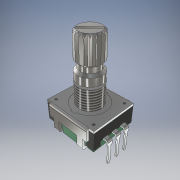
# Autodesk Inventor part: Encoder
Saved by Autodesk Inventor 2018 (Build 220112000, 112)
## iProperties
Created: 2021-02-06
Part Number: Encoder
Material: Všeobecné
Document SubType Name: Modeling
Designer: Jozko Mrkvicka
Density: 1 g/cm^3
Appearance: Výchozí
Author: Jozko Mrkvicka
Autodesk Inventor part; units mm, degrees
sketch "Náčrt1" plane through (0, 0, 0) normal (0, 1, 0) x (-1, 0, 0)
  line L0 (0, 0) -> (11.43, 0)
  line L1 (11.43, 0) -> (11.43, -13.335)
  line L2 (11.43, -13.335) -> (0, -13.335)
  line L3 (0, -13.335) -> (0, 0)
  dimension "d0" = 11.43
  dimension "d1" = 13.335
  constraints: 8 end point, 2 parallel, 1 horizontal, 1 perpendicular
  measures "d0" distance of L1.end L2.end
  measures "d1" distance of L0.end L1.end
extrude "Vysunutí1" add sketch "Náčrt1" along normal blind 3.175
sketch "Náčrt2" plane through (0, 3.175, 0) normal (0, 1, 0) x (1, 0, 0)
  line L0 (-11.43, 13.335) -> (-9.525, 13.335)
  line L1 (-9.525, 13.335) -> (-9.525, 12.7)
  line L2 (-9.525, 12.7) -> (-10.795, 12.7)
  line L3 (-10.795, 12.7) -> (-10.795, 11.43)
  line L4 (-10.795, 11.43) -> (-11.43, 11.43)
  line L5 (-11.43, 11.43) -> (-11.43, 13.335)
  line L6 (-11.43, 0) -> (-11.43, 1.905)
  line L7 (-11.43, 1.905) -> (-10.795, 1.905)
  line L8 (-10.795, 1.905) -> (-10.795, 0.635)
  line L9 (-10.795, 0.635) -> (-9.525, 0.635)
  line L10 (-9.525, 0.635) -> (-9.525, 0)
  line L11 (-9.525, 0) -> (-11.43, 0)
  line L12 (0, 0) -> (-1.905, 0)
  line L13 (-1.905, 0) -> (-1.905, 0.635)
  line L14 (-1.905, 0.635) -> (-0.635, 0.635)
  line L15 (-0.635, 0.635) -> (-0.635, 1.905)
  line L16 (-0.635, 1.905) -> (0, 1.905)
  line L17 (0, 1.905) -> (0, 0)
  line L18 (0, 13.335) -> (0, 11.43)
  line L19 (0, 11.43) -> (-0.635, 11.43)
  line L20 (-0.635, 11.43) -> (-0.635, 12.7)
  line L21 (-0.635, 12.7) -> (-1.905, 12.7)
  line L22 (-1.905, 12.7) -> (-1.905, 13.335)
  line L23 (-1.905, 13.335) -> (0, 13.335)
  point P0 (-11.43, 0)
  point P1 (0, 0)
  point P2 (0, 0)
  point P3 (0, 13.335)
  dimension "d4" = 1.905
  dimension "d5" = 0.635
  dimension "d6" = 1.27
  dimension "d7" = 1.27
  dimension "d8" = 1.905
  dimension "d9" = 0.635
  dimension "d10" = 1.27
  dimension "d11" = 1.27
  dimension "d12" = 1.905
  dimension "d13" = 0.635
  dimension "d14" = 1.27
  dimension "d15" = 1.27
  dimension "d16" = 1.905
  dimension "d17" = 0.635
  dimension "d18" = 1.27
  dimension "d19" = 1.27
  constraints: 48 end point, 8 perpendicular, 1 coincident, 1 vertical
  measures "d4" distance of L0.start L0.end
  measures "d5" distance of L0.end L1.end
  measures "d6" distance of L1.end L2.end
  measures "d7" distance of L2.end L3.end
  measures "d8" distance of L6.start L6.end
  measures "d9" distance of L6.end L7.end
  measures "d10" distance of L7.end L8.end
  measures "d11" distance of L8.end L9.end
  measures "d12" distance of L12.start L12.end
  measures "d13" distance of L12.end L13.end
  measures "d14" distance of L13.end L14.end
  measures "d15" distance of L14.end L15.end
  measures "d16" distance of L18.start L18.end
  measures "d17" distance of L18.end L19.end
  measures "d18" distance of L19.end L20.end
  measures "d19" distance of L20.end L21.end
extrude "Vysunutí2" add sketch "Náčrt2" along normal blind 1.27
sketch "Náčrt3" plane through (0, 3.175, 0) normal (0, 1, 0) x (1, 0, 0)
  line L0 (-11.43, 11.43) -> (-11.43, 1.905) projected
  line L1 (-10.795, 0.635) -> (-0.635, 0.635)
  line L2 (-0.635, 12.7) -> (-10.795, 12.7)
  line L3 (-11.43, 4.445) -> (-11.43, 8.89)
  line L4 (0, 8.89) -> (0, 4.445)
  line L5 (0, 4.445) -> (-0.635, 4.445)
  line L6 (-10.795, 4.445) -> (-11.43, 4.445)
  line L7 (-11.43, 8.89) -> (-10.795, 8.89)
  line L8 (-0.635, 8.89) -> (0, 8.89)
  line L9 (-10.795, 12.7) -> (-10.795, 8.89)
  line L10 (-10.795, 4.445) -> (-10.795, 0.635)
  line L11 (-0.635, 0.635) -> (-0.635, 4.445)
  line L12 (-0.635, 8.89) -> (-0.635, 12.7)
  point P0 (0, 0)
  point P1 (-5.715, 6.6675)
  dimension "d22" = 4.445
  constraints: 24 end point, 10 parallel, 4 perpendicular, 3 horizontal, 1 point on line
  measures "d22" distance of L3.start L3.end
extrude "Vysunutí3" add sketch "Náčrt3" along normal blind 2.54
ref_plane "Pracovní rovina1" through (-10.795, 3.175, -3.175) normal (0, 1, 0) x (1, 0, 0)
split_face "Rozdělit1"
sketch "Náčrt4" plane through (0, 5.715, 0) normal (0, 1, 0) x (1, 0, 0)
  line L0 (-0.635, 4.445) -> (-0.635, 1.905) projected
  line L1 (-0.635, 4.445) -> (-0.635, 1.905)
  line L2 (-10.795, 1.905) -> (-10.795, 4.445)
  line L3 (-10.795, 11.43) -> (-10.795, 8.89)
  line L4 (-0.635, 11.1125) -> (-0.635, 9.2075)
  line L5 (-10.795, 9.2075) -> (-10.795, 11.1125)
  line L6 (-0.635, 4.1275) -> (-0.635, 2.2225)
  line L7 (-10.795, 2.2225) -> (-10.795, 4.1275)
  line L8 (-0.635, 11.1125) -> (-2.54, 11.1125)
  line L9 (-2.54, 11.1125) -> (-2.54, 9.2075)
  line L10 (-2.54, 9.2075) -> (-0.635, 9.2075)
  line L11 (-0.635, 9.2075) -> (-0.635, 11.1125)
  line L12 (-0.635, 4.1275) -> (-2.54, 4.1275)
  line L13 (-2.54, 4.1275) -> (-2.54, 2.2225)
  line L14 (-2.54, 2.2225) -> (-0.635, 2.2225)
  line L15 (-0.635, 2.2225) -> (-0.635, 4.1275)
  line L16 (-10.795, 11.1125) -> (-8.89, 11.1125)
  line L17 (-8.89, 11.1125) -> (-8.89, 9.2075)
  line L18 (-8.89, 9.2075) -> (-10.795, 9.2075)
  line L19 (-10.795, 9.2075) -> (-10.795, 11.1125)
  line L20 (-10.795, 4.1275) -> (-8.89, 4.1275)
  line L21 (-8.89, 4.1275) -> (-8.89, 2.2225)
  line L22 (-8.89, 2.2225) -> (-10.795, 2.2225)
  line L23 (-10.795, 2.2225) -> (-10.795, 4.1275)
  point P0 (0, 0)
  point P1 (-5.715, 10.16)
  point P2 (-5.715, 3.175)
  dimension "d26" = 1.905
  dimension "d27" = 1.905
  dimension "d28" = 1.905
  dimension "d29" = 1.905
  dimension "d30" = 1.905
  dimension "d31" = 1.905
  dimension "d32" = 1.905
  constraints: 46 end point, 11 parallel, 4 horizontal, 4 perpendicular, 1 point on line
  measures "d26" distance of L4.start L4.end
  measures "d27" distance of L6.start L6.end
  measures "d28" distance of L10.end L9.end
  measures "d29" distance of L9.end L8.end
  measures "d30" distance of L14.end L13.end
  measures "d31" distance of L17.end L18.end
  measures "d32" distance of L21.end L22.end
extrude "Vysunutí4" cut sketch "Náčrt4" against normal blind 0.635
sketch "Náčrt5" plane through (0, 0, 0) normal (0, -1, 0) x (1, 0, 0)
  line L0 (0, 0) -> (-11.43, 0) projected
  line L1 (-11.43, 0) -> (-11.43, -13.335) projected
  line L2 (-11.43, -13.335) -> (0, -13.335) projected
  line L3 (0, -13.335) -> (0, 0) projected
  line L4 (0, -13.335) -> (-11.43, -13.335)
  line L5 (-11.43, 0) -> (0, 0)
  line L6 (-11.43, -12.065) -> (-12.065, -12.065)
  line L7 (-12.065, -12.065) -> (-12.065, -1.27)
  line L8 (-12.065, -1.27) -> (-11.43, -1.27)
  line L9 (0, -13.335) -> (0, -11.43) projected
  line L10 (0, -12.065) -> (0.635, -12.065)
  line L11 (0.635, -12.065) -> (0.635, -1.27)
  line L12 (0.635, -1.27) -> (0, -1.27)
  line L13 (0, 0) -> (0, -1.27)
  line L14 (0, -12.065) -> (0, -13.335)
  line L15 (-11.43, -13.335) -> (-11.43, -12.065)
  line L16 (-11.43, -1.27) -> (-11.43, 0)
  dimension "d126" = 1.27
  constraints: 24 end point, 7 parallel, 4 perpendicular, 3 horizontal, 3 point on line
  measures "d126" distance between parallel lines of L12 L0
extrude "Vysunutí5" add sketch "Náčrt5" along normal blind 0.635
ref_plane "Pracovní rovina2" through (0.3175, 0, -1.27) normal (0, 1, 0) x (1, 0, 0)
split_face "Rozdělit2"
sketch "Náčrt6" plane through (0, 0, 0) normal (0, 1, 0) x (1, 0, 0)
  line L0 (0, 1.27) -> (0, 0) projected
  line L1 (0.635, 12.065) -> (0, 12.065)
  line L2 (0, 12.065) -> (0, 1.27)
  line L3 (0, 1.27) -> (0.635, 1.27)
  line L4 (0.635, 1.27) -> (0.635, 12.065)
  line L5 (-11.43, 12.065) -> (-11.43, 13.335) projected
  line L6 (-11.43, 1.27) -> (-12.065, 1.27) projected
  line L7 (-11.43, 12.065) -> (-12.065, 12.065)
  line L8 (-12.065, 12.065) -> (-12.065, 1.27)
  line L9 (-12.065, 1.27) -> (-11.43, 1.27)
  line L10 (-11.43, 1.27) -> (-11.43, 12.065)
  constraints: 16 end point, 4 parallel, 2 horizontal, 2 perpendicular
extrude "Vysunutí6" add sketch "Náčrt6" along normal blind 2.54
sketch "Náčrt7" plane through (0, 2.54, 0) normal (0, 1, 0) x (1, 0, 0)
  line L0 (-2.54, 11.1125) -> (-0.635, 11.1125) projected
  line L1 (-0.635, 11.1125) -> (-0.635, 9.2075) projected
  line L2 (-2.54, 4.1275) -> (-0.635, 4.1275) projected
  line L3 (-0.635, 4.1275) -> (-0.635, 2.2225) projected
  line L4 (-10.795, 4.1275) -> (-8.89, 4.1275) projected
  line L5 (-8.89, 2.2225) -> (-10.795, 2.2225) projected
  line L6 (-10.795, 11.1125) -> (-8.89, 11.1125) projected
  line L7 (-8.89, 9.2075) -> (-10.795, 9.2075) projected
  line L8 (0, 9.3962) -> (0.635, 9.3962)
  line L9 (0.635, 9.3962) -> (0.635, 10.9238)
  line L10 (0.635, 10.9238) -> (0, 10.9238)
  line L11 (0, 10.9238) -> (0, 9.3962)
  line L12 (0, 9.3962) -> (0.635, 10.9238) construction
  line L13 (0.635, 9.3962) -> (0, 10.9238) construction
  line L14 (0, 2.4094) -> (0.635, 2.4094)
  line L15 (0.635, 2.4094) -> (0.635, 3.9406)
  line L16 (0.635, 3.9406) -> (0, 3.9406)
  line L17 (0, 3.9406) -> (0, 2.4094)
  line L18 (0, 2.4094) -> (0.635, 3.9406) construction
  line L19 (0.635, 2.4094) -> (0, 3.9406) construction
  line L20 (-11.43, 2.4094) -> (-12.065, 2.4094)
  line L21 (-12.065, 2.4094) -> (-12.065, 3.9406)
  line L22 (-12.065, 3.9406) -> (-11.43, 3.9406)
  line L23 (-11.43, 3.9406) -> (-11.43, 2.4094)
  line L24 (-11.43, 2.4094) -> (-12.065, 3.9406) construction
  line L25 (-12.065, 2.4094) -> (-11.43, 3.9406) construction
  line L26 (-11.43, 9.3962) -> (-12.065, 9.3962)
  line L27 (-12.065, 9.3962) -> (-12.065, 10.9238)
  line L28 (-12.065, 10.9238) -> (-11.43, 10.9238)
  line L29 (-11.43, 10.9238) -> (-11.43, 9.3962)
  line L30 (-11.43, 9.3962) -> (-12.065, 10.9238) construction
  line L31 (-12.065, 9.3962) -> (-11.43, 10.9238) construction
  point P0 (0.3175, 10.16)
  point P1 (0.3175, 3.175)
  point P2 (-11.7475, 3.175)
  point P3 (-11.7475, 10.16)
  constraints: 48 end point, 8 midpoint, 8 parallel, 4 horizontal, 4 perpendicular, 2 point on line
extrude "Vysunutí7" add sketch "Náčrt7" along normal up to surface (3.175 mm away)
sketch "Náčrt8" plane through (0, 3.175, -9.3962) normal (-1, 0, 0) x (0, 0, 1)
  line L0 (-1.5276, 0) -> (-1.5276, 2.54) projected
  line L1 (0.1887, 1.905) -> (-1.7163, 1.905) projected
  line L2 (0, 2.54) -> (-1.5276, 2.54)
  line L3 (-1.5276, 2.54) -> (-1.5276, 1.905)
  line L4 (-1.5276, 1.905) -> (0, 1.905)
  line L5 (0, 1.905) -> (0, 2.54)
  line L6 (7.1737, 1.905) -> (5.2687, 1.905) projected
  line L7 (6.9868, 2.54) -> (5.4555, 2.54) projected
  line L8 (5.4555, 0) -> (5.4555, 2.54) projected
  line L9 (6.9868, 2.54) -> (5.4555, 2.54)
  line L10 (5.4555, 2.54) -> (5.4555, 1.905)
  line L11 (5.4555, 1.905) -> (6.9868, 1.905)
  line L12 (6.9868, 1.905) -> (6.9868, 2.54)
  point P0 (9.3962, -3.175)
  constraints: 16 end point, 4 parallel, 4 point on line, 2 horizontal, 2 perpendicular
extrude "Vysunutí8" add sketch "Náčrt8" along normal blind 1.905
sketch "Náčrt9" plane through (-11.43, 3.175, -3.9406) normal (1, 0, 0) x (0, 0, -1)
  line L0 (-1.5313, 0) -> (-1.5313, 2.54) projected
  line L1 (0.1869, 1.905) -> (-1.7181, 1.905) projected
  line L2 (7.1719, 1.905) -> (5.2669, 1.905) projected
  line L3 (5.4555, 0) -> (5.4555, 2.54) projected
  line L4 (6.9832, 2.54) -> (5.4555, 2.54)
  line L5 (5.4555, 2.54) -> (5.4555, 1.905)
  line L6 (5.4555, 1.905) -> (6.9832, 1.905)
  line L7 (6.9832, 1.905) -> (6.9832, 2.54)
  line L8 (0, -0.635) -> (0, 2.54) projected
  line L9 (0, 2.54) -> (-1.5313, 2.54)
  line L10 (-1.5313, 2.54) -> (-1.5313, 1.905)
  line L11 (-1.5313, 1.905) -> (0, 1.905)
  line L12 (0, 1.905) -> (0, 2.54)
  point P0 (-3.9406, -3.175)
  constraints: 16 end point, 4 parallel, 4 point on line, 2 horizontal, 2 perpendicular
extrude "Vysunutí9" add sketch "Náčrt9" along normal blind 1.905
fillet "Zaoblení1" radius 0.635 6 edges at (-12.065, 5.715, -10.16) (-12.065, 5.715, -3.175) (0.635, 5.715, -3.175) (0.635, 5.715, -10.16) (0.635, -0.635, -6.6675) (-12.065, -0.635, -6.6675)
fillet "Zaoblení2" radius 0.3175 8 edges at (-11.43, 5.08, -3.175) (-11.43, 5.08, -10.16) (0, 5.08, -10.16) (0, 5.08, -3.175) (-9.525, 5.715, -10.16) (-9.525, 5.715, -3.175) (-1.905, 5.715, -3.175) (-1.905, 5.715, -10.16)
sketch "Náčrt10" plane through (0, -0.635, 0) normal (0, -1, 0) x (1, 0, 0)
  circle A0 centre (-10.16, -12.065) radius 0.3175
  circle A1 centre (-10.16, -1.27) radius 0.3175
  circle A2 centre (-1.27, -1.27) radius 0.3175
  circle A3 centre (-1.27, -12.065) radius 0.3175
  line L0 (-10.4775, -6.0325) -> (-10.4775, -7.3025)
  line L1 (-0.9525, -7.3025) -> (-0.9525, -6.0325)
  line L2 (-10.4775, -7.3025) -> (-10.1144, -7.3025)
  line L3 (-1.3156, -7.3025) -> (-0.9525, -7.3025)
  line L4 (-0.9525, -6.0325) -> (-1.3156, -6.0325)
  line L5 (-10.1144, -6.0325) -> (-10.4775, -6.0325)
  arc A4 (-10.1144, -7.3025) -> (-1.3156, -7.3025) centre (-5.715, -6.6675) ccw
  arc A5 (-1.3156, -6.0325) -> (-10.1144, -6.0325) centre (-5.715, -6.6675) ccw
  line L6 (-11.43, -12.065) -> (-11.43, -1.27) projected
  line L7 (-11.43, -13.335) -> (0, -13.335) projected
  line L8 (0, -13.335) -> (0, -12.065) projected
  line L9 (0, -1.27) -> (0, 0) projected
  line L10 (0, 0) -> (-11.43, 0) projected
  dimension "d55" = 0.635
  dimension "d57" = 0.635
  dimension "d59" = 9.525
  dimension "d60" = 1.27
  dimension "d118" = 1.27
  dimension "d119" = 1.27
  dimension "d120" = 1.27
  dimension "d121" = 1.27
  dimension "d122" = 1.27
  dimension "d123" = 1.27
  dimension "d124" = 1.27
  dimension "d125" = 1.27
  constraints: 12 end point, 6 centre point, 5 parallel, 4 point on circle, 2 coincident, 2 horizontal, 2 perpendicular
  measures "d55" diameter of A1
  measures "d57" diameter of A3
  measures "d59" distance of L1.start L0.end
  measures "d60" distance of L0.end L0.start
  measures "d118" distance from line of L7 point (-10.16, -12.065)
  measures "d119" distance from line of L6 point (-10.16, -12.065)
  measures "d120" distance from line of L7 A3.centre
  measures "d121" distance from line of L8 A3.centre
  measures "d122" distance from line of L10 A2.centre
  measures "d123" distance from line of L9 A2.centre
  measures "d124" distance from line of L10 point (-10.16, -1.27)
  measures "d125" distance from line of L6 point (-10.16, -1.27)
extrude "Vysunutí10" cut sketch "Náčrt10" against normal blind 0.0635
sketch "Náčrt11" plane through (0, -0.5715, 0) normal (0, -1, 0) x (1, 0, 0)
  arc A0 (-10.1144, -7.3025) -> (-1.3156, -7.3025) centre (-5.715, -6.6675) ccw projected
  circle A1 centre (-5.715, -6.6675) radius 3.175
  point P0 (0, 0)
  dimension "d63" = 6.35
  constraints: 1 centre point, 1 coincident
  measures "d63" diameter of A1
extrude "Vysunutí11" add sketch "Náčrt11" along normal blind 5.08
sketch "Náčrt12" plane through (-5.715, -5.6515, -6.6675) normal (0, -1, 0) x (1, 0, 0)
  circle A0 centre (0, 0) radius 3.175 projected
  circle A1 centre (0, 0) radius 2.2225
  point P0 (5.715, 6.6675)
  dimension "d66" = 4.445
  constraints: 1 centre point, 1 coincident
  measures "d66" diameter of A1
extrude "Vysunutí12" add sketch "Náčrt12" along normal blind 0.635 contours A1
sketch "Náčrt13" plane through (-5.715, -6.2865, -6.6675) normal (0, -1, 0) x (1, 0, 0)
  circle A0 centre (0, 0) radius 3.175 projected
  circle A1 centre (0, 0) radius 3.175
  point P0 (5.715, 6.6675)
  constraints: 1 centre point, 1 coincident
extrude "Vysunutí14" add sketch "Náčrt13" along normal blind 2.54
chamfer "Zkosení1" distance 0.635 angle 45 1 edges at (-8.89, -8.8265, -6.6675)
sketch "Náčrt14" plane through (-5.715, -8.8265, -6.6675) normal (0, -1, 0) x (1, 0, 0)
  circle A0 centre (0, 0) radius 2.54 projected
  point P0 (5.715, 6.6675)
extrude "Vysunutí15" add sketch "Náčrt14" along normal blind 1.27
sketch "Náčrt15" plane through (-5.715, -10.0965, -6.6675) normal (0, -1, 0) x (1, 0, 0)
  circle A0 centre (0, 0) radius 3.175
  point P0 (5.715, 6.6675)
  point P1 (-2.5087, 0.3973)
  point P2 (-2.5087, -0.3973)
  point P3 (-2.2632, -1.1531)
  point P4 (-2.5087, -0.3973)
  point P5 (-1.7961, -1.7961)
  point P6 (-2.2632, -1.1531)
  point P7 (-1.1531, -2.2632)
  point P8 (-1.7961, -1.7961)
  point P9 (-0.3973, -2.5087)
  point P10 (-1.1531, -2.2632)
  point P11 (0.3973, -2.5087)
  point P12 (-0.3973, -2.5087)
  point P13 (1.1531, -2.2632)
  point P14 (0.3973, -2.5087)
  point P15 (1.7961, -1.7961)
  point P16 (1.1531, -2.2632)
  point P17 (2.2632, -1.1531)
  point P18 (1.7961, -1.7961)
  point P19 (2.5087, -0.3973)
  point P20 (2.2632, -1.1531)
  point P21 (2.5087, 0.3973)
  point P22 (2.5087, -0.3973)
  point P23 (2.2632, 1.1531)
  point P24 (2.5087, 0.3973)
  point P25 (1.7961, 1.7961)
  point P26 (2.2632, 1.1531)
  point P27 (1.1531, 2.2632)
  point P28 (1.7961, 1.7961)
  point P29 (0.3973, 2.5087)
  point P30 (1.1531, 2.2632)
  point P31 (-0.3973, 2.5087)
  point P32 (0.3973, 2.5087)
  point P33 (-1.1531, 2.2632)
  point P34 (-0.3973, 2.5087)
  point P35 (-1.7961, 1.7961)
  point P36 (-1.1531, 2.2632)
  point P37 (-2.2632, 1.1531)
  point P38 (-1.7961, 1.7961)
  point P39 (-2.5087, 0.3973)
  point P40 (-2.2632, 1.1531)
  constraints: 1 centre point, 1 coincident
extrude "Vysunutí17" add sketch "Náčrt15" along normal blind 6.35
chamfer "Zkosení2" distance 0.635 angle 45 2 edges at (-8.89, -16.4465, -6.6675) (-8.89, -10.0965, -6.6675)
sketch "Náčrt16" plane through (-5.715, -16.4465, -6.6675) normal (0, -1, 0) x (1, 0, 0)
  line L0 (5.08, 6.0325) -> (3.81, 6.0325) projected
  line L1 (2.54, 0) -> (3.3297, 0.6582)
  line L2 (3.3297, 0.6582) -> (3.3297, -0.6582)
  line L3 (5.3975, 4.2581) -> (5.3975, 2.7269) projected
  line L4 (2.54, 0) -> (3.3297, -0.6582)
  line L5 (2.4157, 0.7849) -> (2.9633, 1.6549)
  line L6 (2.9633, 1.6549) -> (3.3701, 0.403)
  line L7 (2.4157, 0.7849) -> (3.3701, 0.403)
  line L8 (2.0549, 1.493) -> (2.3069, 2.4896)
  line L9 (2.3069, 2.4896) -> (3.0806, 1.4247)
  line L10 (2.0549, 1.493) -> (3.0806, 1.4247)
  line L11 (1.493, 2.0549) -> (1.4247, 3.0806)
  line L12 (1.4247, 3.0806) -> (2.4896, 2.3069)
  line L13 (1.493, 2.0549) -> (2.4896, 2.3069)
  line L14 (0.7849, 2.4157) -> (0.403, 3.3701)
  line L15 (0.403, 3.3701) -> (1.6549, 2.9633)
  line L16 (0.7849, 2.4157) -> (1.6549, 2.9633)
  line L17 (0, 2.54) -> (-0.6582, 3.3297)
  line L18 (-0.6582, 3.3297) -> (0.6582, 3.3297)
  line L19 (0, 2.54) -> (0.6582, 3.3297)
  line L20 (-0.7849, 2.4157) -> (-1.6549, 2.9633)
  line L21 (-1.6549, 2.9633) -> (-0.403, 3.3701)
  line L22 (-0.7849, 2.4157) -> (-0.403, 3.3701)
  line L23 (-1.493, 2.0549) -> (-2.4896, 2.3069)
  line L24 (-2.4896, 2.3069) -> (-1.4247, 3.0806)
  line L25 (-1.493, 2.0549) -> (-1.4247, 3.0806)
  line L26 (-2.0549, 1.493) -> (-3.0806, 1.4247)
  line L27 (-3.0806, 1.4247) -> (-2.3069, 2.4896)
  line L28 (-2.0549, 1.493) -> (-2.3069, 2.4896)
  line L29 (-2.4157, 0.7849) -> (-3.3701, 0.403)
  line L30 (-3.3701, 0.403) -> (-2.9633, 1.6549)
  line L31 (-2.4157, 0.7849) -> (-2.9633, 1.6549)
  line L32 (-2.54, 0) -> (-3.3297, -0.6582)
  line L33 (-3.3297, -0.6582) -> (-3.3297, 0.6582)
  line L34 (-2.54, 0) -> (-3.3297, 0.6582)
  line L35 (-2.4157, -0.7849) -> (-2.9633, -1.6549)
  line L36 (-2.9633, -1.6549) -> (-3.3701, -0.403)
  line L37 (-2.4157, -0.7849) -> (-3.3701, -0.403)
  line L38 (-2.0549, -1.493) -> (-2.3069, -2.4896)
  line L39 (-2.3069, -2.4896) -> (-3.0806, -1.4247)
  line L40 (-2.0549, -1.493) -> (-3.0806, -1.4247)
  line L41 (-1.493, -2.0549) -> (-1.4247, -3.0806)
  line L42 (-1.4247, -3.0806) -> (-2.4896, -2.3069)
  line L43 (-1.493, -2.0549) -> (-2.4896, -2.3069)
  line L44 (-0.7849, -2.4157) -> (-0.403, -3.3701)
  line L45 (-0.403, -3.3701) -> (-1.6549, -2.9633)
  line L46 (-0.7849, -2.4157) -> (-1.6549, -2.9633)
  line L47 (0, -2.54) -> (0.6582, -3.3297)
  line L48 (0.6582, -3.3297) -> (-0.6582, -3.3297)
  line L49 (0, -2.54) -> (-0.6582, -3.3297)
  line L50 (0.7849, -2.4157) -> (1.6549, -2.9633)
  line L51 (1.6549, -2.9633) -> (0.403, -3.3701)
  line L52 (0.7849, -2.4157) -> (0.403, -3.3701)
  line L53 (1.493, -2.0549) -> (2.4896, -2.3069)
  line L54 (2.4896, -2.3069) -> (1.4247, -3.0806)
  line L55 (1.493, -2.0549) -> (1.4247, -3.0806)
  line L56 (2.0549, -1.493) -> (3.0806, -1.4247)
  line L57 (3.0806, -1.4247) -> (2.3069, -2.4896)
  line L58 (2.0549, -1.493) -> (2.3069, -2.4896)
  line L59 (2.4157, -0.7849) -> (3.3701, -0.403)
  line L60 (3.3701, -0.403) -> (2.9633, -1.6549)
  line L61 (2.4157, -0.7849) -> (2.9633, -1.6549)
  point P0 (0, 0)
  point P1 (5.715, 6.6675)
  point P2 (0, 0)
  dimension "d113" = 360
  constraints: 120 end point, 1 coincident, 1 parallel, 121 other
extrude "Vysunutí18" cut sketch "Náčrt16" against normal blind 6.35 contours L1 L7 L2 L59 L4 | L7 L5 L10 L6 L1 | L1 L6 L2 L7 | L59 L2 L60 L4 | L4 L60 L56 L61 L59 | L1 L2 L6 | L2 L6 L7 | L60 L2 L4 | L59 L60 L2 | L10 L5 L9 L6 | L6 L9 L10 | L10 L8 L13 L9 L5 | L60 L57 L61 L56 | L56 L57 L60 | L61 L57 L53 L58 L56 | L9 L5 L6 | L60 L61 L57 | L13 L8 L12 L9 | L9 L12 L13 | L13 L11 L16 L12 L8 | L58 L54 L50 L55 L53 | L53 L57 L54 L58 | L53 L54 L57 | L12 L8 L9 | L54 L57 L58 | L16 L11 L15 L12 | L12 L15 L16 | L16 L14 L19 L15 L11 | L55 L51 L47 L52 L50 | L50 L54 L51 L55 | L50 L51 L54 | L15 L11 L12 | L51 L54 L55 | L19 L14 L18 L15 | L15 L18 L19 | L19 L17 L22 L18 L14 | L52 L48 L44 L49 L47 | L47 L51 L48 L52 | L47 L48 L51 | L18 L14 L15 | L48 L51 L52 | L22 L17 L21 L18 | L18 L21 L22 | L22 L20 L25 L21 L17 | L49 L45 L41 L46 L44 | L44 L48 L45 L49 | L44 L45 L48 | L21 L17 L18 | L45 L48 L49 | L25 L20 L24 L21 | L21 L24 L25 | L25 L23 L28 L24 L20 | L46 L42 L38 L43 L41 | L41 L45 L42 L46 | L41 L42 L45 | L24 L20 L21 | L42 L45 L46 | L28 L23 L27 L24 | L24 L27 L28 | L28 L26 L31 L27 L23 | L43 L39 L35 L40 L38 | L38 L42 L39 L43 | L38 L39 L42 | L27 L23 L24 | L39 L42 L43 | L31 L26 L30 L27 | L27 L30 L31 | L31 L29 L34 L30 L26 | L40 L36 L32 L37 L35 | L35 L39 L36 L40 | L35 L36 L39 | L30 L26 L27 | L36 L39 L40 | L34 L29 L33 L30 | L30 L33 L34 | L34 L32 L37 L33 L29 | L32 L36 L33 L37 | L32 L33 L36 | L33 L29 L30 | L33 L36 L37
thread "Závit1" size "5-40 UNC" class "2A" standard "ANSI Unified Screw Threads" full length
sketch "Náčrt17" plane through (-5.715, -16.4465, -6.6675) normal (0, -1, 0) x (1, 0, 0)
  arc A0 (2.0549, -1.493) -> (2.4157, -0.7849) centre (0, 0) ccw projected
  line L0 (2.5608, -1.9365) -> (-1.8799, 2.6026)
  line L1 (-1.8799, 2.6026) -> (-2.5608, 1.9365)
  line L2 (-2.5608, 1.9365) -> (1.8799, -2.6026)
  line L3 (1.8799, -2.6026) -> (2.5608, -1.9365)
  line L4 (2.5608, -1.9365) -> (-2.5608, 1.9365) construction
  line L5 (-1.8799, 2.6026) -> (1.8799, -2.6026) construction
  point P0 (5.715, 6.6675)
  dimension "d127" = 0.9525
  dimension "d130" = 6.35
  constraints: 12 end point, 2 midpoint, 2 parallel, 1 perpendicular
  measures "d127" distance of L1.end L0.end
  measures "d130" distance of L0.start L0.end
extrude "Vysunutí19" cut sketch "Náčrt17" against normal blind 6.35
sketch "Náčrt18" plane through (0, 0, -13.335) normal (0, 0, -1) x (-1, 0, 0)
  line L0 (5.08, 3.175) -> (5.08, 2.8575)
  line L1 (5.08, 2.8575) -> (6.35, 2.8575)
  line L2 (6.35, 2.8575) -> (6.35, 3.175)
  line L3 (1.905, 3.175) -> (9.525, 3.175) projected
  line L4 (3.81, 2.8575) -> (2.54, 2.8575)
  line L5 (2.54, 2.8575) -> (2.54, 3.175)
  line L6 (3.81, 3.175) -> (3.81, 2.8575)
  line L7 (8.89, 2.8575) -> (7.62, 2.8575)
  line L8 (7.62, 2.8575) -> (7.62, 3.175)
  line L9 (8.89, 3.175) -> (8.89, 2.8575)
  line L10 (1.905, 3.175) -> (9.525, 3.175) projected
  line L11 (8.89, 3.175) -> (7.62, 3.175)
  line L12 (6.35, 3.175) -> (5.08, 3.175)
  line L13 (3.81, 3.175) -> (2.54, 3.175)
  point P0 (5.715, 3.175)
  point P1 (3.175, 3.175)
  point P2 (8.255, 3.175)
  point P3 (5.715, 3.175)
  dimension "d131" = 1.27
  dimension "d133" = 1.27
  dimension "d134" = 1.27
  dimension "d135" = 2.54
  dimension "d136" = 2.54
  constraints: 24 end point, 6 point on line, 3 collinear, 3 parallel, 2 horizontal, 2 perpendicular, 1 midpoint, 1 other
  measures "d131" distance of L1.end L0.end
  measures "d133" distance of L5.end L6.start
  measures "d134" distance of L8.end L9.start
  measures "d135" distance of point (8.255, 3.175) point (5.715, 3.175)
  measures "d136" distance of point (5.715, 3.175) point (3.175, 3.175)
extrude "Vysunutí20" add sketch "Náčrt18" along normal blind 1.27
sketch "Náčrt19" plane through (0, 3.175, 0) normal (0, 1, 0) x (1, 0, 0)
  line L0 (-2.54, 14.605) -> (-3.81, 14.605)
  line L1 (-3.81, 14.605) -> (-3.81, 14.2875)
  line L2 (-3.81, 14.2875) -> (-2.54, 14.2875)
  line L3 (-2.54, 14.2875) -> (-2.54, 14.605)
  line L4 (-5.08, 14.605) -> (-6.35, 14.605)
  line L5 (-6.35, 14.605) -> (-6.35, 14.2875)
  line L6 (-6.35, 14.2875) -> (-5.08, 14.2875)
  line L7 (-5.08, 14.2875) -> (-5.08, 14.605)
  line L8 (-7.62, 14.605) -> (-8.89, 14.605)
  line L9 (-8.89, 14.605) -> (-8.89, 14.2875)
  line L10 (-8.89, 14.2875) -> (-7.62, 14.2875)
  line L11 (-7.62, 14.2875) -> (-7.62, 14.605)
  point P0 (0, 0)
  dimension "d139" = 0.3175
  dimension "d142" = 0.3175
  dimension "d143" = 0.3175
  constraints: 24 end point, 6 parallel, 3 horizontal, 3 perpendicular
  measures "d139" distance of L1.end L0.end
  measures "d142" distance of L4.end L5.end
  measures "d143" distance of L8.end L9.end
extrude "Vysunutí21" add sketch "Náčrt19" along normal blind 1.27
sketch "Náčrt20" plane through (0, 4.445, 0) normal (0, 1, 0) x (1, 0, 0)
  line L0 (-7.62, 14.605) -> (-8.89, 14.605) projected
  line L1 (-8.5725, 14.2875) -> (-7.9375, 14.2875)
  line L2 (-7.9375, 14.2875) -> (-7.9375, 14.605)
  line L3 (-7.9375, 14.605) -> (-8.5725, 14.605)
  line L4 (-8.5725, 14.605) -> (-8.5725, 14.2875)
  line L5 (-8.5725, 14.2875) -> (-7.9375, 14.605) construction
  line L6 (-7.9375, 14.2875) -> (-8.5725, 14.605) construction
  line L7 (-6.35, 14.2875) -> (-5.08, 14.2875) projected
  line L8 (-6.0325, 14.605) -> (-5.3975, 14.605)
  line L9 (-5.3975, 14.605) -> (-5.3975, 14.2875)
  line L10 (-5.3975, 14.2875) -> (-6.0325, 14.2875)
  line L11 (-6.0325, 14.2875) -> (-6.0325, 14.605)
  line L12 (-6.0325, 14.605) -> (-5.3975, 14.2875) construction
  line L13 (-5.3975, 14.605) -> (-6.0325, 14.2875) construction
  line L14 (-2.54, 14.605) -> (-3.81, 14.605) projected
  line L15 (-3.4925, 14.2875) -> (-2.8575, 14.2875)
  line L16 (-2.8575, 14.2875) -> (-2.8575, 14.605)
  line L17 (-2.8575, 14.605) -> (-3.4925, 14.605)
  line L18 (-3.4925, 14.605) -> (-3.4925, 14.2875)
  line L19 (-3.4925, 14.2875) -> (-2.8575, 14.605) construction
  line L20 (-2.8575, 14.2875) -> (-3.4925, 14.605) construction
  point P0 (0, 0)
  point P1 (-8.255, 14.4463)
  point P2 (-5.715, 14.4463)
  point P3 (-3.175, 14.4463)
  dimension "d144" = 0.635
  dimension "d145" = 0.635
  dimension "d146" = 0.635
  constraints: 36 end point, 6 midpoint, 6 parallel, 3 horizontal, 3 perpendicular, 3 point on line
  measures "d144" distance of L3.end L2.end
  measures "d145" distance of L9.end L10.end
  measures "d146" distance of L17.end L16.end
extrude "Vysunutí22" add sketch "Náčrt20" along normal blind 5.08
sketch "Náčrt22" plane through (-9.525, 3.175, -0.635) normal (0, 0, 1) x (1, 0, 0)
  line L0 (7.62, 0) -> (0, 0) projected
  line L1 (7.62, 0) -> (6.985, 0)
  line L2 (6.985, 0) -> (5.715, 0)
  line L3 (5.715, 0) -> (5.715, 0.3175)
  line L4 (5.715, 0.3175) -> (6.985, 0.3175)
  line L5 (6.985, 0.3175) -> (6.985, 0)
  line L6 (0, 0) -> (0.635, 0)
  line L7 (0.635, 0) -> (1.905, 0)
  line L8 (1.905, 0) -> (1.905, 0.3175)
  line L9 (1.905, 0.3175) -> (0.635, 0.3175)
  line L10 (0.635, 0.3175) -> (0.635, 0)
  point P0 (9.525, -3.175)
  dimension "d157" = 0.635
  dimension "d158" = 1.27
  dimension "d159" = 0.3175
  dimension "d160" = 0.635
  dimension "d161" = 1.27
  dimension "d162" = 0.3175
  constraints: 20 end point, 4 parallel, 2 horizontal, 2 perpendicular, 2 point on line
  measures "d157" distance of L0.start L1.end
  measures "d158" distance of L3.end L4.end
  measures "d159" distance of L2.end L3.end
  measures "d160" distance of L0.end L6.end
  measures "d161" distance of L9.end L8.end
  measures "d162" distance of L8.end L7.end
extrude "Vysunutí24" add sketch "Náčrt22" along normal blind 1.905
sketch "Náčrt23" plane through (-3.81, 3.4925, -0.635) normal (0, 1, 0) x (1, 0, 0)
  line L0 (0, -0.635) -> (0, -1.905) projected
  line L1 (1.27, -1.905) -> (0, -1.905)
  line L2 (0, -1.905) -> (0, -1.5875)
  line L3 (0, -1.5875) -> (1.27, -1.5875)
  line L4 (1.27, -1.5875) -> (1.27, -1.905)
  line L5 (-5.08, -1.905) -> (-3.81, -1.905) projected
  line L6 (-5.08, -0.635) -> (-5.08, -1.905) projected
  line L7 (-3.81, -1.905) -> (-5.08, -1.905)
  line L8 (-5.08, -1.905) -> (-5.08, -1.5875)
  line L9 (-5.08, -1.5875) -> (-3.81, -1.5875)
  line L10 (-3.81, -1.5875) -> (-3.81, -1.905)
  point P0 (3.81, -0.635)
  dimension "d165" = 0.3175
  constraints: 16 end point, 4 parallel, 3 point on line, 2 horizontal, 2 perpendicular
  measures "d165" distance of L1.end L2.end
extrude "Vysunutí25" add sketch "Náčrt23" along normal blind 1.27
sketch "Náčrt24" plane through (-3.81, 4.7625, -0.635) normal (0, 1, 0) x (1, 0, 0)
  line L0 (0, -1.905) -> (1.27, -1.905) projected
  line L1 (0.9525, -1.5875) -> (0.3175, -1.5875)
  line L2 (0.3175, -1.5875) -> (0.3175, -1.905)
  line L3 (0.3175, -1.905) -> (0.9525, -1.905)
  line L4 (0.9525, -1.905) -> (0.9525, -1.5875)
  line L5 (0.9525, -1.5875) -> (0.3175, -1.905) construction
  line L6 (0.3175, -1.5875) -> (0.9525, -1.905) construction
  line L7 (-5.08, -1.905) -> (-3.81, -1.905) projected
  line L8 (-4.1275, -1.5875) -> (-4.7625, -1.5875)
  line L9 (-4.7625, -1.5875) -> (-4.7625, -1.905)
  line L10 (-4.7625, -1.905) -> (-4.1275, -1.905)
  line L11 (-4.1275, -1.905) -> (-4.1275, -1.5875)
  line L12 (-4.1275, -1.5875) -> (-4.7625, -1.905) construction
  line L13 (-4.7625, -1.5875) -> (-4.1275, -1.905) construction
  point P0 (3.81, -0.635)
  point P1 (0.635, -1.7463)
  point P2 (-4.445, -1.7463)
  dimension "d168" = 0.635
  dimension "d169" = 0.635
  constraints: 24 end point, 4 midpoint, 4 parallel, 2 horizontal, 2 perpendicular, 2 point on line
  measures "d168" distance of L3.end L2.end
  measures "d169" distance of L10.end L9.end
extrude "Vysunutí26" add sketch "Náčrt24" along normal up to surface (4.7625 mm away)
chamfer "Zkosení3" distance 0.3175 angle 45 10 edges at (-2.54, 4.7625, 1.1113) (-3.81, 4.7625, 1.1113) (-8.89, 4.7625, 1.1113) (-7.62, 4.7625, 1.1113) (-8.89, 4.445, -14.4463) (-7.62, 4.445, -14.4463) (-6.35, 4.445, -14.4463) (-5.08, 4.445, -14.4463) (-3.81, 4.445, -14.4463) (-2.54, 4.445, -14.4463)
fillet "Zaoblení3" radius 0.3175 10 edges at (-8.5725, 9.525, -14.4463) (-7.9375, 9.525, -14.4463) (-6.0325, 9.525, -14.4463) (-5.3975, 9.525, -14.4463) (-3.4925, 9.525, -14.4463) (-2.8575, 9.525, -14.4463) (-2.8575, 9.525, 1.1113) (-3.4925, 9.525, 1.1113) (-7.9375, 9.525, 1.1113) (-8.5725, 9.525, 1.1113)
fillet "Zaoblení4" radius 0.508 5 edges at (-8.255, 2.8575, -14.605) (-5.715, 2.8575, -14.605) (-3.175, 2.8575, -14.605) (-8.255, 3.175, 1.27) (-3.175, 3.175, 1.27)
fillet "Zaoblení5" radius 0.254 5 edges at (-3.175, 3.4925, 0.9525) (-8.255, 3.4925, 0.9525) (-8.255, 3.175, -14.2875) (-5.715, 3.175, -14.2875) (-3.175, 3.175, -14.2875)
ref_plane "Pracovní rovina3" through (-8.89, 2.8575, -13.335) normal (0, 0, -1) x (-1, 0, 0)
split_face "Rozdělit3"
